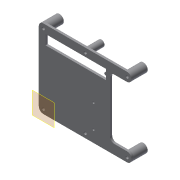
# Autodesk Inventor part: cellSTORM_v5_Electronicbox_midlayer
Saved by Autodesk Inventor 2019 (Build 230136000, 136)
## iProperties
Created: 2020-05-04
Part Number: cellSTORM_v5_Electronicbox_midlayer
Material: Generic
Document SubType Name: Modeling
Designer: diederichbenedict
Density: 1 g/cm^3
Appearance: Default
Author: diederichbenedict
Autodesk Inventor part; units mm, degrees
ref_plane "YZ Plane" through (0, 0, 0) normal (1, 0, 0) x (0, 1, 0)
ref_plane "XZ Plane" through (0, 0, 0) normal (0, 1, 0) x (-1, 0, 0)
ref_plane "Work Plane1" through (0, 0, 15) normal (0, 0, 1) x (1, 0, 0)
sketch "Sketch1" plane through (0, 0, 15) normal (0, 0, 1) x (1, 0, 0)
  circle A0 centre (0, 64) radius 1.4 projected
  circle A1 centre (0, 0) radius 1.4 projected
  circle A2 centre (38.4621, 0) radius 1.4 projected
  circle A3 centre (76.9242, 0) radius 1.4 projected
  circle A4 centre (76.9242, 64) radius 1.4 projected
  circle A5 centre (38.4621, 64) radius 1.4 projected
  circle A6 centre (-0.5, 56.5) radius 1.375 projected
  circle A7 centre (-0.5, 7.5) radius 1.375 projected
  circle A8 centre (57.5, 7.5) radius 1.375 projected
  circle A9 centre (57.5, 56.5) radius 1.375 projected
  line L0 (0, 68) -> (76.9242, 68) projected
  arc A10 (80.9242, 64) -> (76.9242, 68) centre (76.9242, 64) ccw projected
  line L1 (80.9242, 64) -> (80.9242, 0) projected
  arc A11 (76.9242, -4) -> (80.9242, 0) centre (76.9242, 0) ccw projected
  line L2 (76.9242, -4) -> (0, -4) projected
  arc A12 (-4, 0) -> (0, -4) centre (0, 0) ccw projected
  line L3 (-4, 0) -> (-4, 64) projected
  arc A13 (0, 68) -> (-4, 64) centre (0, 64) ccw projected
  line L4 (57.5, 60.619) -> (2.1636, 60.619)
  line L5 (2.1636, 60.619) -> (2.1636, 51.644)
  line L6 (2.1636, 51.644) -> (57.5, 51.644)
  line L7 (57.5, 51.644) -> (57.5, 60.619)
  line L8 (80.9242, 59.8893) -> (61.2665, 59.8893)
  line L9 (61.2665, 59.8893) -> (61.2665, 4.7989)
  line L10 (61.2665, 4.7989) -> (80.9242, 4.7989)
  line L11 (80.9242, 4.7989) -> (80.9242, 59.8893)
  point P0 (0, 0)
  constraints: 16 end point, 4 parallel, 2 horizontal, 2 perpendicular, 1 point on line
extrude "Extrusion1" add sketch "Sketch1" against normal blind 2 contours A6 | A7 | A8 | A9 L7 | L7 A9 | L0 A10 L1 L8 L9 L10 A11 L2 A12 L3 A13
sketch "Sketch2" plane through (0, 0, 13) normal (0, 0, -1) x (-1, 0, 0)
  circle A0 centre (-38.4621, 0) radius 2.9 projected
  circle A1 centre (-38.4621, 64) radius 2.9 projected
  circle A2 centre (0, 0) radius 1.4 projected
  circle A3 centre (-38.4621, 0) radius 1.4 projected
  circle A4 centre (-76.9242, 0) radius 1.4 projected
  circle A5 centre (-76.9242, 64) radius 1.4 projected
  circle A6 centre (-38.4621, 64) radius 1.4 projected
  circle A7 centre (0, 64) radius 1.4 projected
  circle A8 centre (-76.9242, 0) radius 4
  circle A9 centre (-76.9242, 64) radius 4
  circle A10 centre (0, 64) radius 4
  circle A11 centre (0, 0) radius 4
  point P0 (0, 0)
  constraints: 4 centre point, 8 other
ref_plane "Work Plane2" through (-3.375, 53.625, 0) normal (0, 0, 1) x (1, 0, 0)
extrude "Extrusion2" add sketch "Sketch2" along normal up to surface (13 mm away)
fillet "Fillet1" radius 4 4 edges at (61.2665, 4.7989, 14) (61.2665, 59.8893, 14) (80.9242, 59.8893, 14) (80.9242, 4.7989, 14)
sketch "Sketch3" plane through (0, 0, 15) normal (0, 0, 1) x (1, 0, 0)
  circle A0 centre (46, 6.6021) radius 1.05 projected
  line L0 (48, 30.0021) -> (-9, 30.0021) projected
  line L1 (-9, 30.0021) -> (-9, 4.6021) projected
  line L2 (-9, 4.6021) -> (48, 4.6021) projected
  line L3 (48, 4.6021) -> (48, 30.0021) projected
  circle A1 centre (-1, 27.9021) radius 1.05 projected
  circle A2 centre (46, 6.6021) radius 1.05 projected
  circle A3 centre (46, 28.0021) radius 1.05 projected
  circle A4 centre (-0.5, 7.5) radius 1.375 projected
  line L4 (43.458, 3.7531) -> (1.4128, 3.7531)
  line L5 (1.4128, 3.7531) -> (1.4128, 8.2423)
  line L6 (1.4128, 8.2423) -> (43.458, 8.2423)
  line L7 (43.458, 8.2423) -> (43.458, 3.7531)
  line L8 (43.458, 31.4547) -> (0.5917, 31.4547)
  line L9 (0.5917, 31.4547) -> (0.5917, 25.5421)
  line L10 (0.5917, 25.5421) -> (43.458, 25.5421)
  line L11 (43.458, 25.5421) -> (43.458, 31.4547)
  point P0 (0, 0)
  constraints: 16 end point, 4 parallel, 2 horizontal, 2 perpendicular, 1 point on line
extrude "Extrusion3" cut sketch "Sketch3" against normal through all contours A0 | L11 L10 L9 L0 | L0 L9 L8 L11 | L7 L4 L5 L2 | L2 L5 L6 L7 | A3
body "Solid1"
